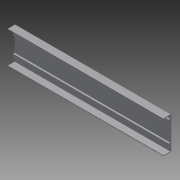
# Autodesk Inventor part: KR45H-340-Protected Cover
Saved by Autodesk Inventor 2011 SP1 (Build 150282100, 282)
## iProperties
Created: 2013-10-24
Part Number: KR45H-340-Protected Cover
Catalog Web Link: www.cadenas.de
Description: LM Guide Actuator - Protected Cover-KR
Vendor: THK
Document SubType Name: Modeling
Designer: PARTuser1
Manufacturer: THK
Density: 1 g/cm^3
Category: PARTsolutions
Company: THK
Title: KR45H-340-Protected Cover
Author: Cadenas PARTsolutions
Comments: KR
PSOL_IDENT_0: {$CADENAS_DATA\23d-libs\thk\lm_guide_actuator\type_kr\parts\lm_g_a_kr_pc.prj},223 {VTYP=3D},{NB=KR45
PSOL_IDENT_1: H-340-Protected Cover},{LINA=KR45H-340-Protected Cover},{NN=LM Guide Actuator - Protected Cover},{DA
PSOL_IDENT_2: TE=17.05.2010 06:32:41},{GEOMDATE=14.02.2008 10:19:00},{VERSION=},{LINEID=60},{LINESUBID=-1},{WBVAR=
PSOL_IDENT_3: LM}  {NB=KR45H-340-Protected Cover},{LINA=KR45H-340-Protected Cover},{KT=DUMMY},{ORDER=KR45H},{TYPE=
PSOL_IDENT_4: 6.000},{LM=340}
CNS_NT: KR
CNS_NB: KR45H-340-Protected Cover
CNS_NBSYN: $ORDER.-$LM.-Protected Cover
CNS_LINA: KR45H-340-Protected Cover
CNS_ORDER: KR45H
CNS_TYPE: 6.000
CNS_LM: 340
SUPPLIER: THK
ARTICLENO: KR45H-340-Protected Cover
BOMINFO: KR45H-340-Protected Cover
CREATOR: CADENAS GmbH
Autodesk Inventor part; units mm, degrees
sketch "Sketch_1" plane through (0, 0, 0) normal (1, 0, 0) x (0, 1, 0)
  line L0 (16, 38.5) -> (0.5, 38.5)
  arc A0 (0.5, 38.5) -> (0, 38) centre (0.5, 38) ccw
  line L1 (0, 38) -> (0, 36.5)
  line L2 (0, 36.5) -> (15.75, 36.5)
  line L3 (15.75, 36.5) -> (15.75, 29.5)
  line L4 (15.75, 29.5) -> (12, 29.5)
  line L5 (12, 29.5) -> (12, 18.5)
  line L6 (12, 18.5) -> (15.75, 18.5)
  line L7 (15.75, 18.5) -> (15.75, -18.5)
  line L8 (15.75, -18.5) -> (12, -18.5)
  line L9 (12, -18.5) -> (12, -29.5)
  line L10 (12, -29.5) -> (15.75, -29.5)
  line L11 (15.75, -29.5) -> (15.75, -36.5)
  line L12 (15.75, -36.5) -> (0, -36.5)
  line L13 (0, -36.5) -> (0, -38)
  arc A1 (0, -38) -> (0.5, -38.5) centre (0.5, -38) ccw
  line L14 (0.5, -38.5) -> (16, -38.5)
  arc A2 (16, -38.5) -> (18, -36.5) centre (16, -36.5) ccw
  line L15 (18, -36.5) -> (18, 36.5)
  arc A3 (18, 36.5) -> (16, 38.5) centre (16, 36.5) ccw
  constraints: 32 end point, 8 point on circle, 4 centre point
extrude "Extrusion1" add sketch "Sketch_1" along normal blind 365
sketch "Sketch_3" plane through (6, 0, 0) normal (1, 0, 0) x (0, 0, -1)
  line L0 (-24, 19.95) -> (-24, 18)
  line L1 (-24, 18) -> (-27.8, 18)
  line L2 (-27.8, 18) -> (-27.8, 19.95)
  line L3 (-27.8, 19.95) -> (-24, 19.95)
  line L4 (-24, 19.95) -> (-24, 18)
  constraints: 10 end point
revolve "Revolution1" add sketch "Sketch_3" angle 360 about axis through (6, 19.95, 24) along (0, 1, 0)
pattern_linear "Rectangular Pattern1" count 2 spacing 353.5 along (1, 0, 0) count 2 spacing 48 along (0, 0, -1) of "Revolution1"
ref_plane "pc_body_XY" through (6, 12, 0) normal (1, 0, 0) x (0, 0, -1)
ref_plane "pc_body_YZ" through (6, 12, 0) normal (0, 0, -1) x (0, 1, 0)
ref_plane "pc_body_ZX" through (6, 12, 0) normal (0, 1, 0) x (1, 0, 0)
body "Solid1"
